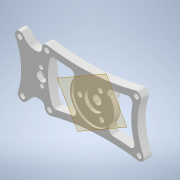
# Autodesk Inventor part: AdapterLplateV2
Saved by Autodesk Inventor 2022 (Build 260153070, 153G)
## iProperties
Created: 2021-11-18
Part Number: AdapterLplateV2
Material: Generic
Document SubType Name: Modeling
Designer: a laptop
Density: 1 g/cm^3
Appearance: Default
Author: a laptop
Autodesk Inventor part; units mm, degrees
ref_plane "YZ Plane" through (0, 0, 0) normal (1, 0, 0) x (0, 1, 0)
ref_plane "XZ Plane" through (0, 0, 0) normal (0, 1, 0) x (-1, 0, 0)
ref_plane "XY Plane" through (0, 0, 0) normal (0, 0, 1) x (1, 0, 0)
ref_plane "Work Plane1" through (5.9765, -10.4058, 6.6) normal (0, 0, 1) x (-0.4980434, 0.8671521, 0)
sketch "Sketch1" plane through (5.9765, -10.4058, 6.6) normal (0, 0, 1) x (-0.4980434, 0.8671521, 0)
  circle A0 centre (12, 0) radius 13
  circle A1 centre (12, 0) radius 12 construction
  circle A2 centre (26.4998, 28.8715) radius 9 construction
  circle A3 centre (22.0316, 31.1155) radius 1.25
  circle A4 centre (30.968, 26.6275) radius 1.25
  circle A5 centre (26.4998, 28.8715) radius 5 construction
  line L0 (22.0316, 31.1155) -> (30.968, 26.6275) construction
  circle A6 centre (23.807, 23.5097) radius 1.1 construction
  circle A7 centre (29.1926, 34.2333) radius 1.1 construction
  line L1 (29.1926, 34.2333) -> (23.807, 23.5097) construction
  circle A8 centre (10.2943, 32.2543) radius 1.55 projected
  circle A9 centre (18.0361, 47.6695) radius 1.55 projected
  circle A10 centre (46.6323, 33.3079) radius 1.55 projected
  circle A11 centre (38.8905, 17.8928) radius 1.55 projected
  arc A12 (37.5217, 15.1672) -> (40.2594, 20.6183) centre (38.8905, 17.8928) ccw projected
  arc A13 (46.5873, 30.2583) -> (46.9025, 36.3459) centre (46.6323, 33.3079) ccw projected
  arc A14 (20.3116, 49.7004) -> (15.6168, 45.8122) centre (18.0361, 47.6695) ccw projected
  arc A15 (11.6631, 34.9799) -> (8.9254, 29.5288) centre (10.2943, 32.2543) ccw projected
  arc A16 (11.6631, 34.9799) -> (15.6083, 35.9802) centre (13.0582, 37.7578) ccw projected
  arc A17 (15.8352, 36.3056) -> (15.6168, 45.8122) centre (9.2305, 40.9097) ccw projected
  line L2 (15.8352, 36.3056) -> (15.6083, 35.9802) projected
  arc A18 (20.3116, 49.7004) -> (46.9025, 36.3459) centre (50.4846, 76.6292) ccw projected
  arc A19 (46.5873, 30.2583) -> (38.8314, 24.7565) centre (46.4684, 22.2081) ccw projected
  arc A20 (38.7058, 24.3802) -> (40.2594, 20.6183) centre (41.6545, 23.3962) ccw projected
  line L3 (38.7058, 24.3802) -> (38.8314, 24.7565) projected
  circle A21 centre (-15.3995, -18.9061) radius 1.55
  circle A22 centre (13.1968, -33.2677) radius 1.55
  line L4 (24.2558, 24.4033) -> (-1.1013, -26.0869) construction
  line L5 (-15.3995, -18.9061) -> (-1.1013, -26.0869) construction
  line L6 (-1.1013, -26.0869) -> (13.1968, -33.2677) construction
  line L7 (10.2943, 32.2543) -> (-15.3995, -18.9061) construction
  arc A23 (15.9224, -34.6365) -> (16.1496, -34.0315) centre (13.1968, -33.2677) ccw
  arc A24 (10.9212, -35.2986) -> (-15.6696, -21.9441) centre (-19.2518, -62.2274) ccw
  arc A25 (-17.7754, -16.9937) -> (-15.6696, -21.9441) centre (-15.3995, -18.9061) ccw
  arc A26 (10.9212, -35.2986) -> (15.9224, -34.6365) centre (13.1968, -33.2677) ccw
  circle A27 centre (26.4998, 28.8715) radius 3 projected
  arc A28 (-17.7754, -16.9937) -> (7.3415, 33.0181) centre (-121.2282, 66.2752) ccw
  line L8 (38.8905, 17.8928) -> (13.1968, -33.2677) construction
  arc A29 (41.2665, 15.9803) -> (16.1496, -34.0315) centre (144.7193, -67.2886) ccw
  point P0 (26.4998, 28.8715)
  dimension "d0" = 1
  dimension "d1" = 10
  dimension "d2" = 2.5
  dimension "d3" = 2.5
  dimension "d4" = 3.1
  dimension "d5" = 3.1
  dimension "d9" = 1.5
  dimension "d12" = 57.25
  dimension "d13" = 3.05
  constraints: 18 point on circle, 15 end point, 12 centre point, 8 tangent, 6 coincident, 4 perpendicular, 3 point on line, 2 collinear, 2 midpoint
  measures "d0" radial gap between concentric circles of A0 A1
  measures "d1" diameter of A5
  measures "d2" diameter of A3
  measures "d3" diameter of A4
  measures "d4" diameter of A21
  measures "d5" diameter of A22
  measures "d9" radial gap between concentric circles of A23 A22
  measures "d12" distance of L7.start L5.start
  measures "d13" distance of A21.centre A25.start
ref_plane "Work Plane2" through (-16.4293, -16.4293, 5.4) normal (0, 0, -1) x (-0.4980434, 0.8671521, 0)
ref_plane "Work Plane3" through (-16.4293, -16.4293, 5.4) normal (0, 0, -1) x (-0.4980434, 0.8671521, 0)
extrude "Extrusion2" add sketch "Sketch1" against normal up to surface (1.2 mm away)
sketch "Sketch3" plane through (8.8827, -148.5371, 5.4) normal (0, 0, -1) x (-0.9984369, -0.0558906, 0)
  circle A0 centre (9.567, 148.8013) radius 1.6 projected
  circle A1 centre (-3.933, 141.0071) radius 1.6 projected
  circle A2 centre (-3.933, 156.5956) radius 1.6 projected
  circle A3 centre (0.567, 148.8013) radius 6.25 construction
  arc A4 (27.9823, 129.8198) -> (-27.9823, 129.8198) centre (0, 0) ccw projected
  arc A5 (27.9823, 129.8198) -> (31.675, 132.8013) centre (28.625, 132.8013) ccw projected
  arc A6 (34.3395, 135.878) -> (31.675, 132.8013) centre (34.7835, 132.8013) ccw projected
  line L0 (34.7321, 135.9347) -> (34.3395, 135.878) projected
  arc A7 (43.1295, 131.4729) -> (34.7321, 135.9347) centre (35.8823, 127.9662) ccw projected
  arc A8 (43.1295, 131.4729) -> (48.7111, 133.9234) centre (45.875, 132.8013) ccw projected
  arc A9 (48.7111, 163.6793) -> (48.7111, 133.9234) centre (86.3172, 148.8013) ccw projected
  arc A10 (48.7111, 163.6793) -> (43.1295, 166.1298) centre (45.875, 164.8013) ccw projected
  arc A11 (34.7321, 161.668) -> (43.1295, 166.1298) centre (35.8823, 169.6364) ccw projected
  line L1 (34.3395, 161.7247) -> (34.7321, 161.668) projected
  arc A12 (31.675, 164.8013) -> (34.3395, 161.7247) centre (34.7835, 164.8013) ccw projected
  arc A13 (31.675, 164.8013) -> (27.9823, 167.7829) centre (28.625, 164.8013) ccw projected
  arc A14 (-27.9823, 167.7829) -> (27.9823, 167.7829) centre (0, 297.6027) ccw projected
  arc A15 (-27.9823, 167.7829) -> (-31.4611, 163.6793) centre (-28.625, 164.8013) ccw projected
  arc A16 (-31.4611, 133.9234) -> (-31.4611, 163.6793) centre (-69.0672, 148.8013) ccw projected
  arc A17 (-31.4611, 133.9234) -> (-27.9823, 129.8198) centre (-28.625, 132.8013) ccw projected
  circle A18 centre (0.567, 148.8013) radius 13 construction
  circle A19 centre (32.875, 143.8013) radius 1.25 projected
  circle A20 centre (32.875, 153.8013) radius 1.25 projected
  circle A21 centre (32.875, 148.8013) radius 3 projected
  circle A22 centre (-28.625, 164.8013) radius 1.55 projected
  circle A23 centre (-28.625, 132.8013) radius 1.55 projected
  circle A24 centre (28.625, 164.8013) radius 1.55 projected
  circle A25 centre (45.875, 164.8013) radius 1.55 projected
  circle A26 centre (45.875, 132.8013) radius 1.55 projected
  circle A27 centre (28.625, 132.8013) radius 1.55 projected
  circle A28 centre (0.567, 148.8013) radius 6
  dimension "d17" = 0.25
  constraints: 1 centre point, 1 coincident
  measures "d17" radial gap between concentric circles of A3 A28
extrude "Extrusion3" add sketch "Sketch3" along normal blind 2
sketch "Sketch4" plane through (8.8827, -148.5371, 3.4) normal (0, 0, -1) x (-0.9984369, -0.0558906, 0)
  arc A0 (48.7111, 163.6793) -> (48.7111, 133.9234) centre (86.3172, 148.8013) ccw projected
  arc A1 (48.7111, 163.6793) -> (43.1295, 166.1298) centre (45.875, 164.8013) ccw projected
  arc A2 (34.7321, 161.668) -> (43.1295, 166.1298) centre (35.8823, 169.6364) ccw projected
  line L0 (34.7321, 161.668) -> (34.3395, 161.7247) projected
  arc A3 (31.675, 164.8013) -> (34.3395, 161.7247) centre (34.7835, 164.8013) ccw projected
  arc A4 (31.675, 164.8013) -> (27.9823, 167.7829) centre (28.625, 164.8013) ccw projected
  arc A5 (-27.9823, 167.7829) -> (27.9823, 167.7829) centre (0, 297.6027) ccw projected
  arc A6 (-27.9823, 167.7829) -> (-31.4611, 163.6793) centre (-28.625, 164.8013) ccw projected
  arc A7 (-31.4611, 133.9234) -> (-31.4611, 163.6793) centre (-69.0672, 148.8013) ccw projected
  arc A8 (-31.4611, 133.9234) -> (-27.9823, 129.8198) centre (-28.625, 132.8013) ccw projected
  arc A9 (27.9823, 129.8198) -> (-27.9823, 129.8198) centre (0, 0) ccw projected
  arc A10 (27.9823, 129.8198) -> (31.675, 132.8013) centre (28.625, 132.8013) ccw projected
  arc A11 (34.3395, 135.878) -> (31.675, 132.8013) centre (34.7835, 132.8013) ccw projected
  line L1 (34.3395, 135.878) -> (34.7321, 135.9347) projected
  arc A12 (43.1295, 131.4729) -> (34.7321, 135.9347) centre (35.8823, 127.9662) ccw projected
  arc A13 (43.1295, 131.4729) -> (48.7111, 133.9234) centre (45.875, 132.8013) ccw projected
  circle A14 centre (9.567, 148.8013) radius 1.6 projected
  circle A15 centre (-3.933, 156.5956) radius 1.6 projected
  circle A16 centre (32.875, 143.8013) radius 1.25 projected
  circle A17 centre (32.875, 153.8013) radius 1.25 projected
  circle A18 centre (32.875, 148.8013) radius 3 construction
  circle A19 centre (0.567, 148.8013) radius 6 construction
  circle A20 centre (28.625, 132.8013) radius 1.55 projected
  circle A21 centre (45.875, 132.8013) radius 1.55 projected
  circle A22 centre (45.875, 164.8013) radius 1.55 projected
  circle A23 centre (28.625, 164.8013) radius 1.55 projected
  circle A24 centre (-28.625, 132.8013) radius 1.55 projected
  circle A25 centre (-28.625, 164.8013) radius 1.55 projected
  circle A26 centre (-3.933, 141.0071) radius 1.6 projected
  circle A27 centre (32.875, 148.8013) radius 1.75
  circle A28 centre (0.567, 148.8013) radius 2.75
  point P0 (0.567, 148.8013)
  dimension "d20" = 3.5
  dimension "d21" = 5.5
  constraints: 2 centre point, 2 coincident
  measures "d20" diameter of A27
  measures "d21" diameter of A28
extrude "Extrusion4" add sketch "Sketch4" along normal blind 2
sketch "Sketch5" plane through (8.8827, -148.5371, 1.4) normal (0, 0, -1) x (-0.9984369, -0.0558906, 0)
  circle A0 centre (0.567, 148.8013) radius 2.75 projected
  circle A1 centre (0.567, 148.8013) radius 9
  circle A2 centre (32.875, 153.8013) radius 1.25 projected
  circle A3 centre (32.875, 143.8013) radius 1.25 projected
  circle A4 centre (32.875, 153.8013) radius 1.25 projected
  line L0 (32.875, 153.8013) -> (32.875, 148.8013) construction
  line L1 (28.625, 148.8013) -> (32.875, 148.8013) construction
  line L2 (32.875, 148.8013) -> (37.125, 148.8013) construction
  line L3 (32.875, 148.8013) -> (32.875, 143.8013) construction
  line L4 (37.125, 148.8013) -> (37.125, 153.8013)
  line L5 (37.125, 148.8013) -> (37.125, 143.8013)
  line L6 (28.625, 148.8013) -> (28.625, 153.8013)
  line L7 (28.625, 148.8013) -> (28.625, 143.8013)
  arc A5 (37.125, 153.8013) -> (28.625, 153.8013) centre (32.875, 153.8013) ccw
  arc A6 (28.625, 143.8013) -> (37.125, 143.8013) centre (32.875, 143.8013) ccw
  circle A7 centre (32.875, 148.8013) radius 1.75 projected
  point P0 (0.567, 148.8013)
  dimension "d24" = 18
  dimension "d25" = 3
  constraints: 16 end point, 6 perpendicular, 5 equal length, 4 point on circle, 3 centre point, 2 concentric, 2 vertical, 1 coincident, 1 tangent
  measures "d24" diameter of A1
  measures "d25" radial gap between concentric circles of A5 A2
ref_plane "Work Plane4" through (-15.0057, -15.0057, 0) normal (0, 0, 1) x (0.8789827, -0.4768537, 0)
extrude "Extrusion5" add sketch "Sketch5" along normal up to surface (1.4 mm away)
ref_plane "Work Plane5" through (-15.6324, -15.6324, -7) normal (0, 0, -1) x (-0.66037, 0.7509404, 0)
sketch "Sketch6" plane through (0, 0, 0) normal (0, 0, -1) x (-1, 0, 0)
  circle A0 centre (0, 0) radius 4 construction
  circle A1 centre (0, 0) radius 2.75 projected
  circle A2 centre (0, 0) radius 4.15
  point P0 (0, 0)
  dimension "d30" = 0.15
  constraints: 1 centre point, 1 coincident
  measures "d30" radial gap between concentric circles of A2 A0
extrude "Extrusion6" add sketch "Sketch6" along normal up to surface (7 mm away)
sketch "Sketch7" plane through (8.8827, -148.5371, 1.4) normal (0, 0, -1) x (-0.9984369, -0.0558906, 0)
  circle A0 centre (9.567, 148.8013) radius 2.85
  arc A1 (9.4248, 147.2077) -> (9.4248, 150.395) centre (9.567, 148.8013) ccw projected
  circle A2 centre (-3.933, 141.0071) radius 2.85
  circle A3 centre (-3.933, 156.5956) radius 2.85
  arc A4 (-2.4817, 157.2692) -> (-5.242, 155.6756) centre (-3.933, 156.5956) ccw projected
  arc A5 (-5.242, 141.9271) -> (-2.4817, 140.3334) centre (-3.933, 141.0071) ccw projected
  point P0 (0.567, 148.8013)
  dimension "d31" = 1.25
  constraints: 3 centre point, 3 concentric, 2 equal radius
  measures "d31" radial gap between concentric circles of A0 A1
extrude "Extrusion7" cut sketch "Sketch7" along normal blind 10
sketch "Sketch8" plane through (8.8827, -148.5371, 1.4) normal (0, 0, -1) x (-0.9984369, -0.0558906, 0)
  circle A0 centre (-28.625, 164.8013) radius 3.05
  arc A1 (-27.9823, 167.7829) -> (-31.4611, 163.6793) centre (-28.625, 164.8013) ccw projected
  circle A2 centre (28.625, 132.8013) radius 3.05
  circle A3 centre (28.625, 164.8013) radius 3.05
  circle A4 centre (-28.625, 132.8013) radius 3.05
  arc A5 (-26.7542, 135.2102) -> (-26.7542, 162.3925) centre (-69.0672, 148.8013) ccw
  arc A6 (-31.4611, 133.9234) -> (-31.4611, 163.6793) centre (-69.0672, 148.8013) ccw projected
  arc A7 (-31.4611, 133.9234) -> (-27.9823, 129.8198) centre (-28.625, 132.8013) ccw projected
  arc A8 (31.675, 164.8013) -> (27.9823, 167.7829) centre (28.625, 164.8013) ccw projected
  arc A9 (27.9823, 129.8198) -> (31.675, 132.8013) centre (28.625, 132.8013) ccw projected
  arc A10 (-25.9757, 163.2901) -> (25.9757, 163.2901) centre (0, 297.6027) ccw
  arc A11 (-27.9823, 167.7829) -> (27.9823, 167.7829) centre (0, 297.6027) ccw projected
  arc A12 (25.9757, 134.3126) -> (-25.9757, 134.3126) centre (0, 0) ccw
  arc A13 (27.9823, 129.8198) -> (-27.9823, 129.8198) centre (0, 0) ccw projected
  circle A14 centre (-3.933, 141.0071) radius 2.85
  circle A15 centre (-3.933, 156.5956) radius 2.85
  arc A16 (-6.1444, 154.7977) -> (-1.2703, 157.6118) centre (-3.933, 156.5956) ccw projected
  arc A17 (-1.2703, 139.9909) -> (-6.1444, 142.8049) centre (-3.933, 141.0071) ccw projected
  arc A18 (-20.061, 135.3224) -> (-9.5412, 143.4186) centre (-22.0592, 148.8013) ccw construction
  arc A19 (-6.1444, 154.7977) -> (-6.1444, 142.8049) centre (0.567, 148.8013) ccw projected
  arc A20 (-8.1438, 161.0439) -> (-9.7117, 154.5643) centre (-3.933, 156.5956) ccw
  arc A21 (-9.8865, 158.0361) -> (-12.2629, 161.3521) centre (-12.5043, 158.6695) ccw
  arc A22 (-22.8479, 162.7228) -> (-25.9131, 159.4235) centre (-23.2978, 160.0673) ccw
  arc A23 (-9.5412, 143.4186) -> (-8.1156, 136.5604) centre (-3.933, 141.0071) ccw
  arc A24 (-12.2426, 136.2524) -> (-9.866, 139.5693) centre (-12.4836, 138.935) ccw
  arc A25 (-25.9131, 138.1791) -> (-22.8479, 134.8799) centre (-23.2978, 137.5354) ccw
  arc A26 (-9.7117, 154.5643) -> (-20.061, 162.2802) centre (-22.0592, 148.8013) ccw construction
  arc A27 (-9.5412, 143.4186) -> (-9.7117, 154.5643) centre (-22.0592, 148.8013) ccw
  arc A28 (26.3857, 134.8721) -> (26.3857, 162.7306) centre (-15.8172, 148.8013) ccw
  line L0 (28.625, 153.8013) -> (28.625, 143.8013) projected
  arc A29 (26.9224, 160.9849) -> (23.8624, 162.8986) centre (24.3322, 160.2465) ccw
  arc A30 (23.8624, 134.7041) -> (26.9224, 136.6178) centre (24.3322, 137.3562) ccw
  arc A31 (7.4308, 136.5994) -> (7.4308, 161.0033) centre (0.567, 148.8013) ccw
  circle A32 centre (0.567, 148.8013) radius 13 projected
  arc A33 (13.6617, 161.4852) -> (11.7746, 157.1912) centre (13.9307, 158.8053) ccw
  arc A34 (11.7746, 140.4114) -> (13.6617, 136.1175) centre (13.9307, 138.7974) ccw
  point P0 (0.567, 148.8013)
  point P1 (-10.0319, 141.2738)
  point P2 (-10.0512, 156.3016)
  dimension "d34" = 4
  dimension "d35" = 4
  dimension "d36" = 4
  dimension "d37" = 6.1253
  dimension "d38" = 1
  constraints: 49 point on circle, 22 centre point, 13 equal radius, 11 tangent, 10 concentric, 3 vertical alignment, 33 other
  measures "d34" radial gap between concentric circles of A6 A5
  measures "d37" radius of A20
  measures "d38" radial gap between concentric circles of A32 A31
extrude "Extrusion8" cut sketch "Sketch8" against normal blind 10 contours A10 A21 A20 A32 A23 A24 A12 A25 A5 A22 | A29 A28 A30 A12 A34 A31 A33 A10
body "Solid2"
